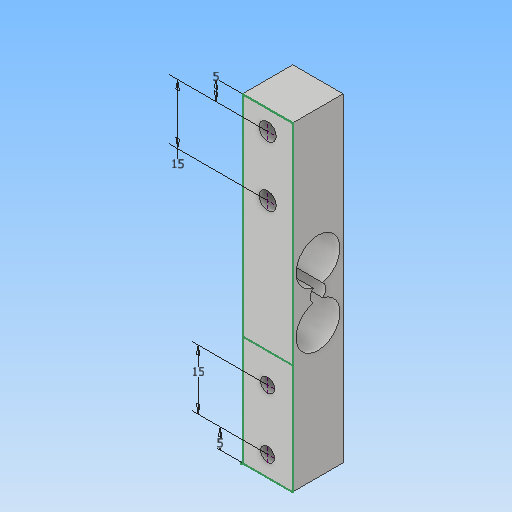
# Autodesk Inventor part: belka_tensometryczna
Saved by Autodesk Inventor 2017 (Build 210142000, 142)
## iProperties
Created: 2017-11-03
Part Number: belka_tensometryczna
Material: Ogólny
Document SubType Name: Modeling
Designer: Kuba01
Density: 1 g/cm^3
Appearance: Domyślna
Author: Kuba01
Autodesk Inventor part; units mm, degrees
ref_plane "YZ Plane" through (0, 0, 0) normal (1, 0, 0) x (0, 1, 0)
ref_plane "XZ Plane" through (0, 0, 0) normal (0, 1, 0) x (-1, 0, 0)
ref_plane "XY Plane" through (0, 0, 0) normal (0, 0, 1) x (1, 0, 0)
sketch "Szkic1" plane through (0, 0, 0) normal (0, 0, 1) x (1, 0, 0)
  point P0 (0, 0)
sketch "Szkic2" plane through (0, 0, 0) normal (0, 1, 0) x (-1, 0, 0)
  line L0 (0, 0) -> (-12.6, 0)
  line L1 (-12.6, 0) -> (-12.6, 12.6)
  line L2 (-12.6, 12.6) -> (0, 12.6)
  line L3 (0, 12.6) -> (0, 0)
  dimension "d0" = 12.6
  dimension "d1" = 12.6
  constraints: 8 end point, 2 parallel, 1 horizontal, 1 perpendicular
  measures "d0" distance of L1.end L2.end
  measures "d1" distance of L0.end L1.end
extrude "Wyciągnięcie proste1" add sketch "Szkic2" along normal blind 80
sketch "Szkic3" plane through (12.6, 0, 12.6) normal (1, 0, 0) x (0, 0, -1)
  line L0 (12.6, 0) -> (0, 0) projected
  line L1 (12.6, 0) -> (12.6, 80) projected
  line L2 (0, 80) -> (12.6, 80) projected
  line L3 (0, 0) -> (0, 80) projected
  arc A0 (5.1341, 38.375) -> (7.4659, 38.375) centre (6.3, 33) ccw
  arc A1 (7.4659, 41.625) -> (5.1341, 41.625) centre (6.3, 47) ccw
  arc A2 (5.1341, 41.625) -> (5.1341, 38.375) centre (6.3, 40) ccw
  arc A3 (7.4659, 38.375) -> (7.4659, 41.625) centre (6.3, 40) ccw
  dimension "d5" = 11
  dimension "d6" = 33
  dimension "d7" = 11
  dimension "d8" = 33
  constraints: 8 point on circle, 4 centre point
  measures "d5" diameter of A0
  measures "d6" distance from line of A0.centre L0
  measures "d7" diameter of A1
  measures "d8" distance from line of A1.centre L2
extrude "Wyciągnięcie proste2" cut sketch "Szkic3" against normal blind 80 contours A2 A1 A3 A0
sketch "Szkic4" plane through (0, 0, 12.6) normal (0, 0, 1) x (1, 0, 0)
  line L0 (12.6, 27.5) -> (0, 27.5) projected
  line L1 (12.6, 0) -> (0, 0) projected
  line L2 (12.6, 0) -> (12.6, 80) projected
  line L3 (0, 80) -> (12.6, 80) projected
  line L4 (0, 0) -> (0, 80) projected
  point P0 (6.3, 5)
  point P1 (6.3, 20)
  point P2 (6.3, 60)
  point P3 (6.3, 75)
  dimension "d11" = 5
  dimension "d12" = 15
  dimension "d13" = 5
  dimension "d15" = 15
  measures "d11" distance from line of point (6.3, 5) L1
  measures "d12" distance of point (6.3, 20) point (6.3, 5)
  measures "d13" distance from line of point (6.3, 75) L3
  measures "d15" distance of point (6.3, 60) point (6.3, 75)
hole "Otwór1" at (6.3, 5, 12.6) at (6.3, 20, 12.6) direction (0, 0, -1) diameter 3.5 end through all
hole "Otwór2" at (6.3, 60, 12.6) at (6.3, 75, 12.6) direction (0, 0, -1) diameter 4.3 end through all
